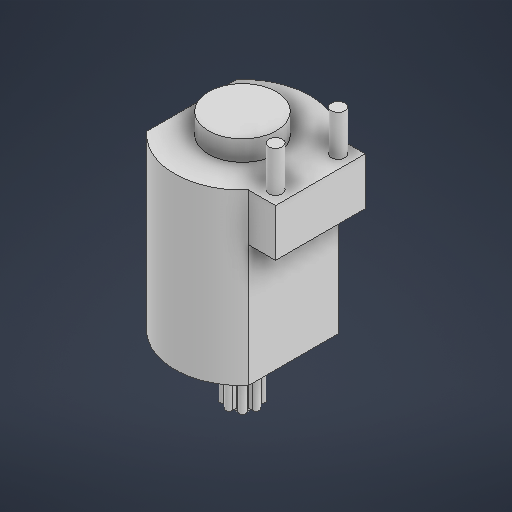
# Autodesk Inventor part: motor
Saved by Autodesk Inventor 2025.2 (Build 292293000, 293)
## iProperties
Created: 2025-05-21
Part Number: motor
Material: Generic
Document SubType Name: Modeling
Designer: klawy
Density: 1 g/cm^3
Appearance: Default
Author: klawy
Autodesk Inventor part; units mm, degrees
ref_plane "YZ Plane" through (0, 0, 0) normal (1, 0, 0) x (0, 1, 0)
ref_plane "XZ Plane" through (0, 0, 0) normal (0, 1, 0) x (-1, 0, 0)
ref_plane "XY Plane" through (0, 0, 0) normal (0, 0, 1) x (1, 0, 0)
sketch "Sketch1" plane through (0, 0, 0) normal (0, 1, 0) x (-1, 0, 0)
  line L0 (7.5, 6.6144) -> (7.5, -6.6144)
  line L1 (-7.5, -6.6144) -> (-7.5, 6.6144)
  arc A0 (-7.5, -6.6144) -> (7.5, -6.6144) centre (0, 0) ccw
  arc A1 (7.5, 6.6144) -> (-7.5, 6.6144) centre (0, 0) ccw
  dimension "d1" = 15
  dimension "d2" = 7.5
  dimension "d3" = 10
  dimension "d4" = 10
  constraints: 4 end point, 4 point on circle, 2 centre point, 2 vertical, 1 coincident
  measures "d1" distance between parallel lines of L1 L0
  measures "d2" distance from line of point (0, 0) L1
  measures "d3" radius of A1
  measures "d4" radius of A0
extrude "Extrusion1" add sketch "Sketch1" along normal blind 25
sketch "Sketch2" plane through (0, 0, 0) normal (0, -1, 0) x (1, 0, 0)
  circle A0 centre (0, 0) radius 3
  dimension "d7" = 6
  constraints: 1 centre point, 1 coincident
  measures "d7" diameter of A0
extrude "Extrusion2" add sketch "Sketch2" along normal blind 2
sketch "Sketch3" plane through (0, -2, 0) normal (0, -1, 0) x (1, 0, 0)
  circle A0 centre (0, 0) radius 2
  dimension "d10" = 4
  constraints: 1 centre point, 1 coincident
  measures "d10" diameter of A0
extrude "Extrusion3" add sketch "Sketch3" along normal blind 3
sketch "Sketch4" plane through (0, 25, 0) normal (0, 1, 0) x (1, 0, 0)
  circle A0 centre (0, 0) radius 2 projected
  circle A1 centre (0, 0) radius 5
  dimension "d13" = 10
  constraints: 1 centre point, 1 coincident
  measures "d13" diameter of A1
extrude "Extrusion4" add sketch "Sketch4" along normal blind 3 contours A0 | A1
sketch "Sketch5" plane through (7.5, 0, 6.6144) normal (1, 0, 0) x (0, 0, -1)
  line L0 (0, 0) -> (0, 25) projected
  line L1 (13.2288, 0) -> (13.2288, 25) projected
  line L2 (0, 25) -> (13.2288, 25)
  line L3 (13.2288, 25) -> (13.2288, 18)
  line L4 (13.2288, 18) -> (0, 18)
  line L5 (0, 18) -> (0, 25)
  point P0 (6.6144, 0)
  point P1 (0, 18)
  dimension "d16" = 7
  constraints: 8 end point, 2 parallel, 1 horizontal, 1 perpendicular, 1 point on line
  measures "d16" distance between parallel lines of L2 L4
extrude "Extrusion5" add sketch "Sketch5" along normal blind 4
sketch "Sketch7" plane through (0, -5, 0) normal (0, -1, 0) x (1, 0, 0)
  circle A0 centre (0, 0) radius 2.5
  dimension "d21" = 5
  constraints: 1 centre point, 1 coincident
  measures "d21" diameter of A0
extrude "Extrusion7" add sketch "Sketch7" along normal blind 4
sketch "Sketch8" plane through (0, -9, 0) normal (0, -1, 0) x (1, 0, 0)
  circle A0 centre (0, 0) radius 1.5
  circle A1 centre (0, 0) radius 2.5
  line L0 (-0.5, 1) -> (0.5, 1)
  line L1 (0.5, 1) -> (0.5, 2)
  line L2 (0.5, 2) -> (-0.5, 2) construction
  line L3 (-0.5, 2) -> (-0.5, 1)
  line L4 (-0.5, 1) -> (0.5, 2) construction
  line L5 (0.5, 1) -> (-0.5, 2) construction
  circle A2 centre (0, 2) radius 0.5
  line L6 (-0.3536, 1.0607) -> (-1.0607, 1.7678)
  line L7 (-1.0607, 1.7678) -> (-1.7678, 1.0607) construction
  line L8 (-1.0607, 0.3536) -> (-1.0607, 1.7678) construction
  circle A3 centre (-1.4142, 1.4142) radius 0.5
  line L9 (-1.7678, 1.0607) -> (-1.0607, 0.3536)
  line L10 (-1, 0.5) -> (-2, 0.5)
  line L11 (-2, 0.5) -> (-2, -0.5) construction
  line L12 (-1, -0.5) -> (-2, 0.5) construction
  circle A4 centre (-2, 0) radius 0.5
  line L13 (-2, -0.5) -> (-1, -0.5)
  line L14 (-1.0607, -0.3536) -> (-1.7678, -1.0607)
  line L15 (-1.7678, -1.0607) -> (-1.0607, -1.7678) construction
  line L16 (-0.3536, -1.0607) -> (-1.7678, -1.0607) construction
  circle A5 centre (-1.4142, -1.4142) radius 0.5
  line L17 (-1.0607, -1.7678) -> (-0.3536, -1.0607)
  line L18 (-0.5, -1) -> (-0.5, -2)
  line L19 (-0.5, -2) -> (0.5, -2) construction
  line L20 (0.5, -1) -> (-0.5, -2) construction
  circle A6 centre (0, -2) radius 0.5
  line L21 (0.5, -2) -> (0.5, -1)
  line L22 (0.3536, -1.0607) -> (1.0607, -1.7678)
  line L23 (1.0607, -1.7678) -> (1.7678, -1.0607) construction
  line L24 (1.0607, -0.3536) -> (1.0607, -1.7678) construction
  circle A7 centre (1.4142, -1.4142) radius 0.5
  line L25 (1.7678, -1.0607) -> (1.0607, -0.3536)
  line L26 (1, -0.5) -> (2, -0.5)
  line L27 (2, -0.5) -> (2, 0.5) construction
  line L28 (1, 0.5) -> (2, -0.5) construction
  circle A8 centre (2, 0) radius 0.5
  line L29 (2, 0.5) -> (1, 0.5)
  line L30 (1.0607, 0.3536) -> (1.7678, 1.0607)
  line L31 (1.7678, 1.0607) -> (1.0607, 1.7678) construction
  line L32 (0.3536, 1.0607) -> (1.7678, 1.0607) construction
  circle A9 centre (1.4142, 1.4142) radius 0.5
  line L33 (1.0607, 1.7678) -> (0.3536, 1.0607)
  point P0 (0, 1.5)
  point P1 (-1.0607, 1.0607)
  point P2 (-1.5, 0)
  point P3 (-1.0607, -1.0607)
  point P4 (0, -1.5)
  point P5 (1.0607, -1.0607)
  point P6 (1.3536, -0.6464)
  point P7 (1.7678, -1.7678)
  point P8 (0, 2.5)
  point P9 (0.5, 1.4142)
  point P10 (1.0607, -1.7678)
  point P11 (0.6464, -1.3536)
  point P12 (0.5, -1.4142)
  point P13 (0, -2.5)
  point P14 (-0.5, -1.4142)
  point P15 (-0.6464, -1.3536)
  point P16 (-1.7678, -1.7678)
  point P17 (-1.7678, -1.0607)
  point P18 (-1.3536, -0.6464)
  point P19 (-1.4142, -0.5)
  point P20 (-2.5, 0)
  point P21 (-1.4142, 0.5)
  point P22 (-1.3536, 0.6464)
  point P23 (-1.7678, 1.7678)
  point P24 (-0.6464, 1.3536)
  point P25 (-0.5, 1.4142)
  point P26 (1.5, 0)
  point P27 (1.0607, 1.0607)
  point P28 (0.6464, 1.3536)
  point P29 (1.7678, 1.7678)
  point P30 (1.3536, 0.6464)
  point P31 (1.4142, 0.5)
  point P32 (2.5, 0)
  point P33 (1.4142, -0.5)
  dimension "d24" = 3
  dimension "d25" = 5
  dimension "d26" = 1
  dimension "d29" = 360
  constraints: 68 end point, 3 midpoint, 2 coincident, 2 parallel, 1 centre point, 1 horizontal, 1 perpendicular, 1 vertical alignment, 117 other
  measures "d25" diameter of A1
  measures "d26" distance of L2.end L1.end
extrude "Extrusion8" cut sketch "Sketch8" against normal blind 4 contours A0 L30 A9 A1 A8 L29 | L26 A8 A1 A7 L25 A0 | A9 L33 A0 L1 A2 A1 | A1 A6 L21 A0 L22 A7 | A2 L3 A0 L6 A3 A1 | A1 A5 L17 A0 L18 A6 | A3 L9 A0 L10 A4 A1 | A1 A4 L13 A0 L14 A5
sketch "Sketch9" plane through (0, -9, 0) normal (0, -1, 0) x (1, 0, 0)
  circle A0 centre (0, 0) radius 1
  dimension "d33" = 2
  constraints: 1 centre point, 1 coincident
  measures "d33" diameter of A0
extrude "Extrusion9" add sketch "Sketch9" along normal blind 1
fillet "Fillet1" radius 0.25 1 edges at (-1, -10, 0)
sketch "Sketch10" plane through (0, 25, 0) normal (0, 1, 0) x (1, 0, 0)
  circle A0 centre (9.5, 4.6144) radius 1
  circle A1 centre (9.5, -4.6144) radius 1
  line L0 (11.5, 6.6144) -> (11.5, -6.6144) projected
  line L1 (7.5, 6.6144) -> (11.5, 6.6144) projected
  line L2 (7.5, -6.6144) -> (11.5, -6.6144) projected
  point P0 (0, 0)
  dimension "d37" = 2
  dimension "d38" = 2
  dimension "d39" = 2
  dimension "d40" = 2
  dimension "d41" = 2
  dimension "d42" = 2
  constraints: 2 centre point
  measures "d37" diameter of A1
  measures "d38" diameter of A0
  measures "d39" distance from line of L0 A0.centre
  measures "d40" distance from line of L1 A0.centre
  measures "d41" distance from line of A1.centre L2
  measures "d42" distance from line of A1.centre L0
extrude "Extrusion10" add sketch "Sketch10" along normal blind 6
body "Solid1"
